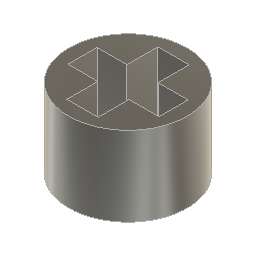
cylindrical_lp v10 (Autodesk Fusion 360 archive; units mm, degrees)
design "mx_stem"
Autodesk Fusion 360 part; units mm, degrees
sketch "Sketch1" plane through (0, 0, 0) normal (0, 0, 1) x (1, 0, 0)
  line L0 (-0.725, 2.115) -> (0.725, 2.115)
  line L1 (0.725, 2.115) -> (0.725, -2.115)
  line L2 (0.725, -2.115) -> (-0.725, -2.115)
  line L3 (-0.725, -2.115) -> (-0.725, 2.115)
  line L4 (-0.725, 2.115) -> (0.725, -2.115) construction
  line L5 (0.725, 2.115) -> (-0.725, -2.115) construction
  line L6 (-2.115, 0.675) -> (2.115, 0.675)
  line L7 (2.115, 0.675) -> (2.115, -0.675)
  line L8 (2.115, -0.675) -> (-2.115, -0.675)
  line L9 (-2.115, -0.675) -> (-2.115, 0.675)
  line L10 (-2.115, 0.675) -> (2.115, -0.675) construction
  line L11 (2.115, 0.675) -> (-2.115, -0.675) construction
  circle A0 centre (0, 0) radius 2.75
  dimension "d21" = 1.45
  dimension "d22" = 4.23
  dimension "d23" = 4.23
  dimension "d24" = 1.35
  dimension "d25" = 5.5
  constraint horizontal L0
  constraint perpendicular L0 L1
  constraint parallel L0 L2
  constraint parallel L1 L3
  constraint coincident L4 A0.centre
  constraint coincident L5 A0.centre
  constraint coincident A0.centre origin
  constraint horizontal L6
  constraint perpendicular L6 L7
  constraint parallel L6 L8
  constraint parallel L7 L9
  constraint coincident L10 A0.centre
  constraint coincident L11 A0.centre
  measures "d21" distance of L1.end L2.end
  measures "d22" distance of L0.end L1.end
  measures "d23" distance of L7.end L8.end
  measures "d24" distance of L6.end L7.end
  measures "d25" diameter of A0
extrude "Extrude1" add sketch "Sketch1" against normal blind 3.7
chamfer "Chamfer1" distance 0.235 angle 65 4 edges at (-2.115, 0, -3.7) (2.115, 0, -3.7) (0, -2.115, -3.7) (0, 2.115, -3.7) measured on face at (-1.6186, -1.0735, -3.7) measured on face at (-1.6186, -1.0735, -3.7) measured on face at (-1.6186, -1.0735, -3.7) measured on face at (-1.6186, -1.0735, -3.7)
chamfer "Chamfer2" distance 0.0889 angle 80 8 edges at (0.725, 1.5125, -3.7) (1.5375, 0.675, -3.7) (1.5375, -0.675, -3.7) (0.725, -1.5125, -3.7) (-0.725, -1.5125, -3.7) (-1.5375, -0.675, -3.7) (-1.5375, 0.675, -3.7) (-0.725, 1.5125, -3.7) measured on face at (-1.0549, 1.725, -3.7) measured on face at (-1.0549, 1.725, -3.7) measured on face at (-1.0549, 1.725, -3.7) measured on face at (-1.0549, 1.725, -3.7) measured on face at (-1.0549, 1.725, -3.7) measured on face at (-1.0549, 1.725, -3.7) measured on face at (-1.0549, 1.725, -3.7) measured on face at (-1.0549, 1.725, -3.7)
equation "width = 5.5 mm"
equation "depth = 5.5 mm"
equation "cross_xy = 4.23 mm"
equation "gap_x = 1.35 mm"
equation "gap_y = 1.45 mm"
equation "height = 3.7 mm"
equation "d13 = -height"
equation "d15 = chamfer_cross"
equation "d16 = chamfer_cross_angle"
equation "d17 = chamfer_gap"
equation "d18 = chamfer_gap_angle"
equation "d21 = gap_y"
equation "d22 = cross_xy"
equation "d23 = cross_xy"
equation "d24 = gap_x"
equation "d25 = width"
equation "chamfer_cross_angle = 65 deg"
equation "chamfer_cross = 0.235 mm"
equation "chamfer_gap_angle = 80 deg"
equation "chamfer_gap = 0.088857 mm"
